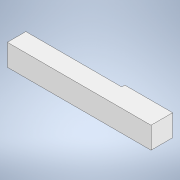
# Autodesk Inventor part: Key--Lowest
Saved by Autodesk Inventor 2021 (Build 250183000, 183)
## iProperties
Created: 2021-03-17
Part Number: Key--Lowest
Material: Generic
Document SubType Name: Modeling
Designer: Tom
Density: 1 g/cm^3
Appearance: White
Author: Tom
Autodesk Inventor part; units mm, degrees
ref_plane "YZ Plane" through (0, 0, 0) normal (1, 0, 0) x (0, 1, 0)
ref_plane "XZ Plane" through (0, 0, 0) normal (0, 1, 0) x (-1, 0, 0)
ref_plane "XY Plane" through (0, 0, 0) normal (0, 0, 1) x (1, 0, 0)
sketch "Sketch1" plane through (0, 0, 0) normal (0, 1, 0) x (-1, 0, 0)
  line L0 (147.6375, -19.05) -> (49.2125, -19.05)
  line L1 (49.2125, -19.05) -> (49.2125, -22.225)
  line L2 (49.2125, -22.225) -> (0, -22.225)
  line L3 (0, -22.225) -> (0, 0)
  line L4 (147.6375, -19.05) -> (147.6375, 0)
  line L5 (147.6375, 0) -> (0, 0)
  dimension "d0" = 22.225
  dimension "d2" = 98.425
  dimension "d8" = 19.05
  dimension "d9" = 147.6375
  constraints: 12 end point, 3 perpendicular, 1 vertical
  measures "d0" distance of L2.end L3.end
  measures "d2" distance of L0.start L0.end
  measures "d8" distance between parallel lines of L0 L5
  measures "d9" distance between parallel lines of L4 L3
extrude "Extrusion1" add sketch "Sketch1" against normal blind 22.225
body "Solid1"
